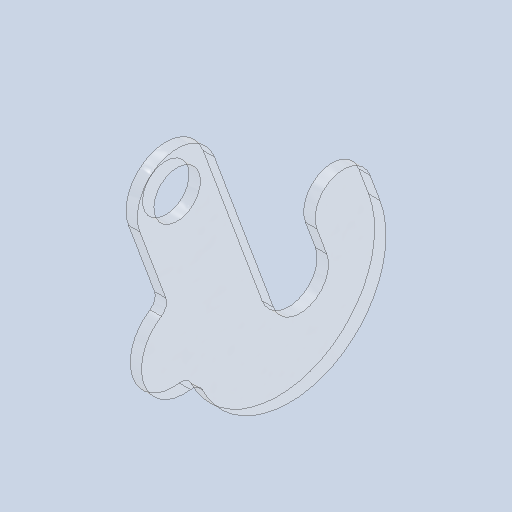
# Autodesk Inventor part: part3
Saved by Autodesk Inventor 2025.2 (Build 292293000, 293)
## iProperties
Created: 2025-02-28
Part Number: part3
Material: アクリル、クリア
Document SubType Name: Modeling
Designer: haruy
Density: 1.19 g/cm^3
Appearance: 透明 - クリア
Author: haruy
Autodesk Inventor part; units mm, degrees
ref_plane "YZ Plane" through (0, 0, 0) normal (1, 0, 0) x (0, 1, 0)
ref_plane "XZ Plane" through (0, 0, 0) normal (0, 1, 0) x (-1, 0, 0)
ref_plane "XY Plane" through (0, 0, 0) normal (0, 0, 1) x (1, 0, 0)
derived "oikon-Sketch-Base.ipt"
sketch "スケッチ1" plane through (100, 0, 0) normal (1, 0, 0) x (0, 1, 0)
  line L0 (0, 0) -> (-50, 0)
  line L1 (-50, 0) -> (-50, -2)
  line L2 (-50, -2) -> (0, -2)
  line L3 (0, -2) -> (0, 0)
  circle A0 centre (-10, -6) radius 4 construction
  circle A1 centre (-10, -6) radius 7
  line L4 (-26, 13) -> (-45, 13)
  line L5 (-45, 13) -> (-45, 2.35)
  line L6 (-45, 2.35) -> (-26, 2.35)
  line L7 (-26, 2.35) -> (-26, 13)
  line L8 (0, 14.6) -> (-50, 14.6)
  line L9 (-50, 14.6) -> (-50, 13)
  line L10 (-50, 13) -> (0, 13)
  line L11 (0, 13) -> (0, 14.6)
  line L12 (0, 36.6) -> (-50, 36.6)
  line L13 (-50, 36.6) -> (-50, 34.6)
  line L14 (-50, 34.6) -> (0, 34.6)
  line L15 (0, 34.6) -> (0, 36.6)
  line L16 (-12.427, 0.5658) -> (-40.5661, -9.8358)
  arc A2 (-34, 2.35) -> (-32, 2.35) centre (-33, 2.35) ccw
  line L17 (-7.573, -12.5658) -> (-35.712, -22.9674)
  line L18 (-40.5661, -9.8358) -> (-35.712, -22.9674)
  line L19 (-35.712, -22.9674) -> (-28.7776, -41.7268)
  arc A3 (-35.712, -22.9674) -> (-32.2448, -32.3471) centre (-33.9784, -27.6572) ccw
  line L20 (-32.2448, -32.3471) -> (-27.555, -30.6135)
  line L21 (-27.555, -30.6135) -> (-26.1339, -34.4579)
  arc A4 (-24.0878, -39.9932) -> (-27.555, -30.6135) centre (-25.8214, -35.3033) ccw
  line L22 (-24.0878, -39.9932) -> (-28.7776, -41.7268)
  arc A5 (-40.5661, -9.8358) -> (-28.7776, -41.7268) centre (-34.6719, -25.7813) ccw
  line L23 (0, 0) -> (5, 0)
  line L24 (5, 0) -> (5, -2)
  line L25 (5, -2) -> (0, -2)
  line L26 (0, -2) -> (0, 0)
  line L27 (0, 36.6) -> (5, 36.6)
  line L28 (5, 36.6) -> (5, 34.6)
  line L29 (5, 34.6) -> (0, 34.6)
  line L30 (0, 34.6) -> (0, 36.6)
  line L31 (-50, 36.6) -> (-55, 36.6)
  line L32 (-55, 36.6) -> (-55, 34.6)
  line L33 (-55, 34.6) -> (-50, 34.6)
  line L34 (-50, 34.6) -> (-50, 36.6)
  line L35 (-50, 0) -> (-55, 0)
  line L36 (-55, 0) -> (-55, -2)
  line L37 (-55, -2) -> (-50, -2)
  line L38 (-50, -2) -> (-50, 0)
  circle A6 centre (-10, -6) radius 4.1
  arc A7 (-26.4966, -4.635) -> (-40.5661, -9.8358) centre (-33.5313, -7.2354) ccw
  point P0 (-14.1989, 2.35)
  point P1 (-12.427, 0.5658)
  point P2 (-28.7776, -41.7268)
  point P3 (-22.4439, -2.1076)
  point P4 (-39.8222, -6.7973)
  point P5 (-26.4966, -4.635)
  dimension "d1" = 8.2
  measures "d1" diameter of A6
extrude "押し出し1" add sketch "スケッチ1" along normal blind 2 contours A1 L2 A6 L0 | L0 A1 | A1 L2 L16 L0 | L0 L16 A1 | A1 L2 A6 | A1 L17 L18 L16 L2 | A7 L2 L0 | L0 A7 | A7 L16 L2 | A3 L19 A5 L18 | L20 A4 L22 L19 picked at (-31.1864, -2.8783)
fillet "フィレット4" radius 2 2 edges at (101, -26.4966, -4.635) (101, -40.5661, -9.8358)
